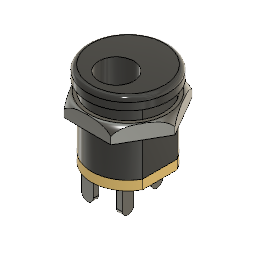
610 DC Jack (Autodesk Fusion 360 design; units mm, degrees)
Autodesk Fusion 360 part; units mm, degrees
sketch "Sketch1" plane through (0, 0, 0) normal (0, 0, 1) x (1, 0, 0)
  circle A0 centre (0, 0) radius 8
  circle A1 centre (0, 0) radius 7
  circle A2 centre (0, -2) radius 3
  dimension "d1" = 16
  dimension "d2" = 14
  dimension "d3" = 6
  dimension "d4" = 2
  measures "d1" diameter of A0
  measures "d2" diameter of A1
  measures "d3" diameter of A2
  measures "d4" distance of A0.centre
extrude "Extrude1" add sketch "Sketch1" along normal blind 1 contours A1 | A2 makes body 1
extrude "Extrude2" add sketch "Sketch1" along normal blind 2 contours A1 bodies 1
sketch "Sketch2" plane through (0, 0, 0) normal (0, 0, 1) x (1, 0, 0)
  circle A0 centre (0, 0) radius 6.25
  line L0 (5.5, -6.25) -> (-5.5, -6.25)
  line L1 (-5.5, -6.25) -> (-5.5, 6.25)
  line L2 (-5.5, 6.25) -> (5.5, 6.25)
  line L3 (5.5, 6.25) -> (5.5, -6.25)
  line L4 (5.5, -6.25) -> (-5.5, 6.25) construction
  line L5 (-5.5, -6.25) -> (5.5, 6.25) construction
  dimension "d10" = 12.5
  dimension "d12" = 12.5
  dimension "d13" = 11
  measures "d10" diameter of A0
extrude "Extrude3" add sketch "Sketch2" against normal blind 12.5 contours A0 L1 L3 bodies 1
sketch "Sketch3" plane through (0, 0, 0) normal (0, 0, 1) x (1, 0, 0)
  line L0 (4.0415, -7) -> (8.0829, 0)
  line L1 (8.0829, 0) -> (4.0415, 7)
  line L2 (4.0415, 7) -> (-4.0415, 7)
  line L3 (-4.0415, 7) -> (-8.0829, 0)
  line L4 (-8.0829, 0) -> (-4.0415, -7)
  line L5 (-4.0415, -7) -> (4.0415, -7)
  circle A0 centre (0, 0) radius 6.25
  dimension "d16" = 7
  dimension "d17" = 12.5
  measures "d16" distance of A0.centre L5
  measures "d17" diameter of A0
extrude "Extrude4" add sketch "Sketch3" against normal blind 2.5 separate body makes body 2
sketch "Sketch4" plane through (0, 0, -12.5) normal (0, 0, -1) x (1, 0, 0)
  arc A0 (5.5, 2.9686) -> (-5.5, 2.9686) centre (0, 0) ccw
  line L0 (-5.5, 2.9686) -> (-5.5, -2.9686)
  arc A1 (-5.5, -2.9686) -> (5.5, -2.9686) centre (0, 0) ccw
  line L1 (5.5, -2.9686) -> (5.5, 2.9686)
  line L2 (-0.5, 0) -> (-3.5, 0)
  line L3 (-3.5, 0) -> (-3.5, 4)
  line L4 (-3.5, 4) -> (-0.5, 4)
  line L5 (-0.5, 4) -> (-0.5, 0)
  line L6 (2, -4) -> (1, -4)
  line L7 (1, -4) -> (1, -2)
  line L8 (1, -2) -> (2, -2)
  line L9 (2, -2) -> (2, -4)
  line L10 (3.5, 4.5) -> (2.5, 4.5)
  line L11 (2.5, 4.5) -> (2.5, 2.5)
  line L12 (2.5, 2.5) -> (3.5, 2.5)
  line L13 (3.5, 2.5) -> (3.5, 4.5)
  circle A2 centre (-2, 1.5) radius 1
  line L14 (-2, 1.5) -> (-2, 0)
  line L15 (-1, 4) -> (-3, 4)
  line L16 (-3, 4) -> (-3, 5)
  line L17 (-3, 5) -> (-1, 5)
  line L18 (-1, 5) -> (-1, 4)
  dimension "d20" = 1
  dimension "d21" = 2
  dimension "d22" = 2
  dimension "d23" = 1
  dimension "d24" = 3
  dimension "d25" = 4
  dimension "d26" = 2
  dimension "d27" = 1.5
  dimension "d40" = 2
  dimension "d41" = 1
  measures "d24" distance of A0.centre
  measures "d25" distance of A0.centre
  measures "d26" diameter of A2
  measures "d27" distance of L2
extrude "Extrude9" cut sketch "Sketch4" against normal blind 1.6 contours A0 L0 A1 L1 | L2 L3 L4 L5 L15 | L4 L15 L16 L17 L18 | L6 L7 L8 L9 | L10 L11 L12 L13 | A2 bodies 1
extrude "Extrude10" add sketch "Sketch4" against normal blind 1.6 separate body contours A0 L0 A1 L1 | L2 L3 L4 L5 L15 | L4 L15 L16 L17 L18 | L6 L7 L8 L9 | L10 L11 L12 L13 | A2 makes body 3
extrude "Extrude5" add sketch "Sketch4" along normal blind 4.5 contours L6 L7 L8 L9 | L10 L11 L12 L13 bodies 1 makes body 4 at (3.5, -3.1667, -14) makes body 5 at (1, 3.3333, -14)
extrude "Extrude6" add sketch "Sketch4" along normal blind 1 contours L2 L3 L4 L5 L15 bodies 4 1 5 makes body 6
fillet "Fillet1" radius 1.5 2 edges at (-0.5, 0, -13) (-3.5, 0, -13) on bodies 6
extrude "Extrude7" add sketch "Sketch4" along normal blind 4.5 contours L4 L15 L16 L17 L18 bodies 4 6 5 1
fillet "Fillet2" radius 1 6 edges at (3, -4.5, -17) (3, -2.5, -17) (1.5, 2, -17) (1.5, 4, -17) (-1, -4.5, -17) (-3, -4.5, -17) on bodies 4 5 6
extrude "Extrude8" cut 1 faces at (0.9661, -2.866, 1) along direction (0, 0, -1) blind 9 on bodies 1 bodies 5 4 6 1
fillet "Fillet3" radius 0.75 1 edges at (-6.5263, -2.5313, 2) on bodies 1
sketch "Sketch5" plane through (0, 0, 0) normal (1, 0, 0) x (0, 1, 0)
  spline S0 degree 5 poles (-6.8, 0) (-6.8774, 0) (-7.0322, -0.0264) (-7.2642, -0.1452) (-7.5682, -0.4337) (-7.9062, -0.8936) (-8.1027, -1.244) (-8.1823, -1.4503) (-8.2, -1.5555) (-8.2, -1.6) knots 0 0 0 0 0 0 0.2 0.4 0.6 0.8 1 1 1 1 1 1
  line L0 (-8.2, -1.2408) -> (-8.2, -1.9592)
  line L1 (-6.2, 0) -> (-7.4, 0)
  line L2 (7, 0) -> (0, 0)
  line L3 (-8.2, -1.6) -> (-8.2, -2.5)
  line L4 (-8.2, -2.5) -> (0, -2.5)
  line L5 (0, -2.5) -> (0, 0)
  line L6 (-6.8, 0) -> (0, 0)
revolve "Revolve1" cut sketch "Sketch5" angle 360 about axis through (0, 0, -2.5) along (0, 0, 1) keep common part bodies 2
move_body "Move1" bodies 2 to x (1, 0, 0) y (0, 1, 0) z (0, 0, 1) at (0, 0, -2)
